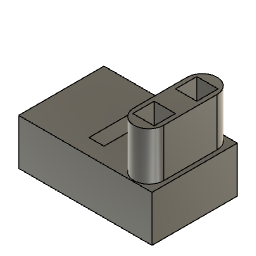
drawing_1 v2 (Autodesk Fusion 360 design; units mm, degrees)
Autodesk Fusion 360 part; units mm, degrees
sketch "Sketch1" plane through (0, 0, 0) normal (0, 0, 1) x (1, 0, 0)
  line L0 (0, 0) -> (-125, 0)
  line L1 (-125, 0) -> (-125, 80)
  line L2 (-125, 80) -> (0, 80)
  line L3 (0, 80) -> (0, 0)
  dimension "d1" = 125
  dimension "d2" = 80
  constraint horizontal L0
  constraint vertical L1
  constraint horizontal L2
  constraint vertical L3
  constraint coincident L0.start L3.end
  measures "d1" distance of L0.start L0.end
  measures "d2" distance of L0.start L2.end
extrude "Extrude1" add sketch "Sketch1" along normal blind 43
sketch "Sketch2" plane through (0, 0, 43) normal (0, 0, 1) x (-1, 0, 0)
  line L0 (0, -80) -> (125, -80)
  line L1 (125, -80) -> (125, 0)
  line L2 (125, 0) -> (0, 0)
  line L3 (0, 0) -> (0, -80)
  line L4 (67, -40) -> (67, -15)
  line L5 (67, -40) -> (67, -65)
  line L6 (67, -15) -> (74, -15)
  line L7 (67, -15) -> (60, -15)
  line L8 (60, -15) -> (60, -65)
  line L9 (74, -15) -> (74, -65)
  line L10 (74, -65) -> (60, -65)
  dimension "d6" = 25
  dimension "d7" = 25
  dimension "d8" = 7
  dimension "d9" = 50
  dimension "d10" = 50
  constraint parallel L4 L5
  constraint perpendicular L4 L6
  constraint perpendicular L4 L7
  constraint perpendicular L6 L8
  constraint perpendicular L6 L9
  measures "d6" distance of L4.start L4.end
  measures "d7" distance of L4.start L5.end
  measures "d8" distance of L4.end L6.end
  measures "d9" distance of L7.end L8.end
  measures "d10" distance of L6.end L9.end
extrude "Extrude2" cut sketch "Sketch2" against normal blind 75 contours L4 L5 L7 L8 L10 | L4 L5 L6 L9 L10
sketch "Sketch3" plane through (0, 0, 43) normal (0, 0, 1) x (-1, 0, 0)
  line L0 (60, -65) -> (60, -15)
  line L1 (60, -15) -> (74, -15)
  line L2 (74, -15) -> (74, -65)
  line L3 (74, -65) -> (60, -65)
  line L4 (0, -80) -> (125, -80)
  line L5 (125, -80) -> (125, 0)
  line L6 (125, 0) -> (0, 0)
  line L7 (0, 0) -> (0, -80)
  line L8 (67, -15) -> (85, -15)
  line L9 (85, -15) -> (85, -65)
  line L10 (85, -65) -> (49, -65)
  line L11 (49, -65) -> (49, -15)
  line L12 (49, -15) -> (67, -15)
  dimension "d13" = 18
  dimension "d14" = 50
  dimension "d15" = 36
  dimension "d16" = 50
  constraint midpoint L1 L8.start
  constraint perpendicular L2 L8
  constraint perpendicular L8 L9
  constraint perpendicular L9 L10
  constraint perpendicular L10 L11
  measures "d13" distance of L8.start L8.end
  measures "d14" distance of L8.end L9.end
  measures "d15" distance of L9.end L10.end
  measures "d16" distance of L10.end L11.end
extrude "Extrude3" cut sketch "Sketch3" against normal blind 8 contours L0 L10 L11 L12 | L2 L8 L9 L10
sketch "Sketch4" plane through (0, 0, 43) normal (0, 0, 1) x (-1, 0, 0)
  line L0 (49, -15) -> (85, -15)
  line L1 (85, -15) -> (85, -65)
  line L2 (85, -65) -> (49, -65)
  line L3 (49, -65) -> (49, -15)
  line L4 (0, -80) -> (125, -80)
  line L5 (125, -80) -> (125, 0)
  line L6 (125, 0) -> (0, 0)
  line L7 (0, 0) -> (0, -80)
  circle A0 centre (109, -40) radius 12.5
  dimension "d20" = 25
  measures "d20" diameter of A0
extrude "Extrude4" cut sketch "Sketch4" against normal blind 27 contours A0
move_body "Move1" bodies 1 to x (1, 0, 0) y (0, -1, 0) z (0, 0, -1) at (0, 65.5278, 86)
sketch "Sketch5" plane through (0, 0, 86) normal (0, 0, 1) x (-1, 0, 0)
  line L0 (60, -50.5278) -> (60, -0.5278)
  line L1 (60, -0.5278) -> (74, -0.5278)
  line L2 (74, -0.5278) -> (74, -50.5278)
  line L3 (74, -50.5278) -> (60, -50.5278)
  line L4 (125, 14.4722) -> (0, 14.4722)
  line L5 (0, 14.4722) -> (0, -65.5278)
  line L6 (0, -65.5278) -> (125, -65.5278)
  line L7 (125, -65.5278) -> (125, 14.4722)
  line L8 (18, -45.5278) -> (28, -45.5278)
  line L9 (28, -45.5278) -> (28, -55.5278)
  line L10 (28, -55.5278) -> (18, -55.5278)
  line L11 (18, -55.5278) -> (18, -45.5278)
  line L12 (18, -5.5278) -> (28, -5.5278)
  line L13 (28, -5.5278) -> (28, 4.4722)
  line L14 (28, 4.4722) -> (18, 4.4722)
  line L15 (18, 4.4722) -> (18, -5.5278)
  line L16 (18, 4.4722) -> (8, 4.4722)
  line L17 (8, 4.4722) -> (8, -15.5278)
  line L18 (8, -15.5278) -> (18, -15.5278)
  line L19 (18, -15.5278) -> (18, 4.4722)
  line L20 (28, -5.5278) -> (18, -5.5278)
  line L21 (18, -5.5278) -> (18, -15.5278)
  line L22 (18, -15.5278) -> (28, -15.5278)
  line L23 (28, -15.5278) -> (28, -5.5278)
  line L24 (18, -55.5278) -> (8, -55.5278)
  line L25 (8, -55.5278) -> (8, -35.5278)
  line L26 (8, -35.5278) -> (18, -35.5278)
  line L27 (18, -35.5278) -> (18, -55.5278)
  line L28 (18, -35.5278) -> (28, -35.5278)
  line L29 (28, -35.5278) -> (28, -45.5278)
  line L30 (28, -45.5278) -> (18, -45.5278)
  line L31 (18, -45.5278) -> (18, -35.5278)
  dimension "d26" = 10
  dimension "d27" = 10
  dimension "d28" = 10
  dimension "d29" = 10
  dimension "d30" = 10
  dimension "d31" = 20
  dimension "d32" = 10
  dimension "d33" = 20
  constraint horizontal L8
  constraint vertical L9
  constraint horizontal L10
  constraint vertical L11
  constraint horizontal L12
  constraint vertical L13
  constraint horizontal L14
  constraint vertical L15
  constraint horizontal L16
  constraint vertical L17
  constraint horizontal L18
  constraint vertical L19
  constraint horizontal L20
  constraint vertical L21
  constraint horizontal L22
  constraint vertical L23
  constraint horizontal L24
  constraint vertical L25
  constraint horizontal L26
  constraint vertical L27
  constraint horizontal L28
  constraint vertical L29
  constraint horizontal L30
  constraint vertical L31
  measures "d26" distance of L8.start L8.end
  measures "d27" distance of L8.start L10.end
  measures "d28" distance of L12.start L12.end
  measures "d29" distance of L12.start L14.end
  measures "d30" distance of L14.end L16.end
  measures "d31" distance of L14.end L18.end
  measures "d32" distance of L10.end L24.end
  measures "d33" distance of L10.end L26.end
sketch "Sketch6" plane through (0, 0, 86) normal (0, 0, 1) x (-1, 0, 0)
sketch "Sketch7" plane through (0, 0, 86) normal (0, 0, 1) x (1, 0, 0)
extrude "Extrude5" cut sketch "Sketch5" against normal blind 70 contours L8 L27 L28 L29 L30 L31 | L8 L9 L10 L11 L27 L30 | L11 L24 L25 L26 L27 L31 | L12 L13 L14 L15 L19 L20 | L15 L16 L17 L18 L19 L21 | L12 L19 L20 L21 L22 L23
sketch "Sketch8" plane through (0, 0, 86) normal (0, 0, 1) x (-1, 0, 0)
  line L0 (8, 4.4722) -> (28, 4.4722)
  line L1 (28, 4.4722) -> (28, -15.5278)
  line L2 (28, -15.5278) -> (8, -15.5278)
  line L3 (8, -15.5278) -> (8, 4.4722)
  line L4 (8, -55.5278) -> (8, -35.5278)
  line L5 (8, -35.5278) -> (28, -35.5278)
  line L6 (28, -35.5278) -> (28, -55.5278)
  line L7 (28, -55.5278) -> (8, -55.5278)
  line L8 (60, -50.5278) -> (60, -0.5278)
  line L9 (60, -0.5278) -> (74, -0.5278)
  line L10 (74, -0.5278) -> (74, -50.5278)
  line L11 (74, -50.5278) -> (60, -50.5278)
  line L12 (125, 14.4722) -> (0, 14.4722)
  line L13 (0, 14.4722) -> (0, -65.5278)
  line L14 (0, -65.5278) -> (125, -65.5278)
  line L15 (125, -65.5278) -> (125, 14.4722)
  line L16 (4, 4.4722) -> (4, -55.5278)
  line L17 (32, -55.5278) -> (32, 4.4722)
  circle A0 centre (18, -50.5278) radius 14
  line L18 (18, 4.4722) -> (18, -0.5278)
  circle A1 centre (18, -0.5278) radius 14
  dimension "d36" = 4
  dimension "d37" = 4
  dimension "d38" = 4
  dimension "d39" = 4
  dimension "d42" = 5
  constraint tangent L17 A0
  constraint midpoint L0 L18.start
  constraint perpendicular L0 L18
  constraint coincident L18.end A1.centre
  constraint tangent L17 A1
  measures "d36" distance of L0.start L16.start
  measures "d37" distance of L4.start L16.end
  measures "d38" distance of L0.end L17.end
  measures "d39" distance of L6.end L17.start
  measures "d42" distance of L18.start L18.end
extrude "Extrude6" add sketch "Sketch8" along normal blind 45 contours L0 L1 L3 A1 | L1 L2 L3 L4 L5 L6 L16 L17 A0 A1 | L4 L6 L7 A0 picked at (11.757, 6.4541) picked at (18.3487, -58.5147)
